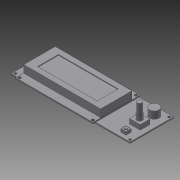
# Autodesk Inventor part: RepRapDiscount_SmartController
Saved by Autodesk Inventor 2014 (Build 180170000, 170)
## iProperties
Created: 2014-10-27
Part Number: RepRapDiscount_SmartController
Material: Generic
Document SubType Name: Modeling
Designer: ThatOtherGuy
Density: 1 g/cm^3
Appearance: Default
Author: ThatOtherGuy
Autodesk Inventor part; units mm, degrees
note: some values were not read from the file. Chosen so that the rebuilt part matches the saved one: direction of "LCD_PCB_Hole".
ref_plane "YZ Plane" through (0, 0, 0) normal (1, 0, 0) x (0, 1, 0)
ref_plane "XZ Plane" through (0, 0, 0) normal (0, 1, 0) x (-1, 0, 0)
ref_plane "XY Plane" through (0, 0, 0) normal (0, 0, 1) x (1, 0, 0)
sketch "Sketch1" plane through (0, 0, 0) normal (0, 0, 1) x (1, 0, 0)
  line L0 (0, 0) -> (150, 0)
  line L1 (150, 0) -> (150, 55)
  line L2 (150, 55) -> (0, 55)
  line L3 (0, 55) -> (0, 0)
  dimension "d0" = 150
  dimension "d1" = 55
  constraints: 8 end point, 2 parallel, 1 horizontal, 1 perpendicular
  measures "d0" distance of L1.end L2.end
  measures "d1" distance of L2.end L0.start
extrude "BackerPCB" add sketch "Sketch1" along normal blind 1.6
sketch "Sketch2" plane through (0, 0, 1.6) normal (0, 0, 1) x (1, 0, 0)
  line L0 (0, 0) -> (150, 0) projected
  line L1 (150, 0) -> (150, 55) projected
  line L2 (150, 55) -> (0, 55) projected
  line L3 (0, 55) -> (0, 0) projected
  point P0 (2.61, 52.265)
  point P1 (147.39, 52.265)
  point P2 (147.39, 2.735)
  point P3 (2.61, 2.735)
  dimension "d4" = 144.78
  dimension "d5" = 49.53
  dimension "d6" = 2.735
  dimension "d7" = 2.61
  dimension "d9" = 2.61
  dimension "d10" = 2.735
  constraints: 2 horizontal alignment, 2 vertical alignment
  measures "d4" distance of point (2.61, 52.265) point (147.39, 52.265)
  measures "d5" distance of point (2.61, 52.265) point (2.61, 2.735)
  measures "d6" distance from line of L2 point (2.61, 52.265)
  measures "d7" distance from line of L3 point (2.61, 52.265)
  measures "d9" distance from line of L1 point (147.39, 52.265)
  measures "d10" distance from line of L0 point (2.61, 2.735)
hole "BackerPCB_Holes" at (2.61, 52.265, 1.6) at (147.39, 52.265, 1.6) at (147.39, 2.735, 1.6) at (2.61, 2.735, 1.6) direction (0, 0, -1) diameter 3 end through all
sketch "Sketch3" plane through (0, 0, 0) normal (0, 0, -1) x (-1, 0, 0)
  line L0 (0, 0) -> (-150, 0) projected
  line L1 (0, 55) -> (0, 0) projected
  line L2 (0, 34.25) -> (-26, 34.25)
  line L3 (-26, 34.25) -> (-26, 7.75)
  line L4 (-26, 7.75) -> (0, 7.75)
  line L5 (0, 7.75) -> (0, 34.25)
  dimension "d18" = 26
  dimension "d19" = 26.5
  dimension "d20" = 7.75
  constraints: 8 end point, 2 parallel, 1 horizontal, 1 perpendicular, 1 point on line
  measures "d18" distance of L2.start L2.end
  measures "d19" distance of L2.end L3.end
  measures "d20" distance between parallel lines of L0 L4
extrude "SDSlot" add sketch "Sketch3" along normal blind 2.75
sketch "Sketch4" plane through (0, 0, 0) normal (0, 0, -1) x (-1, 0, 0)
  line L0 (0, 55) -> (0, 0) projected
  line L1 (-150, 55) -> (0, 55) projected
  circle A0 centre (-13, 43) radius 4.5
  dimension "d23" = 9
  dimension "d24" = 13
  dimension "d25" = 12
  constraints: 1 centre point
  measures "d23" diameter of A0
  measures "d24" distance from line of L0 A0.centre
  measures "d25" distance from line of L1 A0.centre
extrude "ContrastPot" add sketch "Sketch4" along normal blind 7.75
sketch "Sketch5" plane through (0, 0, 0) normal (0, 0, -1) x (-1, 0, 0)
  line L0 (-150, 55) -> (0, 55) projected
  line L1 (-150, 0) -> (-150, 55) projected
  line L2 (-89, 32.5) -> (-68.5, 32.5)
  line L3 (-68.5, 32.5) -> (-68.5, 23.75)
  line L4 (-68.5, 23.75) -> (-89, 23.75)
  line L5 (-89, 23.75) -> (-89, 32.5)
  line L6 (-66.1, 32.5) -> (-45.6, 32.5)
  line L7 (-45.6, 32.5) -> (-45.6, 23.75)
  line L8 (-45.6, 23.75) -> (-66.1, 23.75)
  line L9 (-66.1, 23.75) -> (-66.1, 32.5)
  dimension "d28" = 20.5
  dimension "d29" = 8.75
  dimension "d30" = 2.4
  dimension "d31" = 22.5
  dimension "d32" = 61
  constraints: 16 end point, 4 parallel, 2 equal length, 2 horizontal, 2 perpendicular, 1 collinear
  measures "d28" distance of L2.start L2.end
  measures "d29" distance of L4.end L2.start
  measures "d30" distance between parallel lines of L9 L3
  measures "d31" distance between parallel lines of L0 L2
  measures "d32" distance between parallel lines of L1 L5
extrude "Ribbons" add sketch "Sketch5" along normal blind 9
sketch "Sketch6" plane through (0, 0, 1.6) normal (0, 0, 1) x (1, 0, 0)
  line L0 (150, 0) -> (150, 55) projected
  line L1 (150, 55) -> (0, 55) projected
  circle A0 centre (136.2, 44.5) radius 6
  dimension "d35" = 13.8
  dimension "d36" = 10.5
  dimension "d37" = 12
  constraints: 1 centre point
  measures "d35" distance from line of L0 A0.centre
  measures "d36" distance from line of L1 A0.centre
  measures "d37" diameter of A0
extrude "Piezo" add sketch "Sketch6" along normal blind 9
sketch "Sketch14" plane through (0, 0, 1.6) normal (0, 0, 1) x (1, 0, 0)
  line L0 (0, 0) -> (150, 0) projected
  line L1 (150, 0) -> (150, 55) projected
  line L2 (133.65, 11.35) -> (140, 11.35)
  line L3 (140, 11.35) -> (140, 5)
  line L4 (140, 5) -> (133.65, 5)
  line L5 (133.65, 5) -> (133.65, 11.35)
  dimension "d84" = 6.35
  dimension "d85" = 5
  dimension "d86" = 10
  constraints: 8 end point, 2 parallel, 2 perpendicular, 1 horizontal
  measures "d84" distance of L2.start L2.end
  measures "d85" distance between parallel lines of L0 L4
  measures "d86" distance between parallel lines of L1 L3
extrude "Button_Base" add sketch "Sketch14" along normal blind 4
sketch "Sketch15" plane through (0, 0, 5.6) normal (0, 0, 1) x (1, 0, 0)
  line L0 (140, 11.35) -> (133.65, 11.35) projected
  line L1 (133.65, 11.35) -> (133.65, 5) projected
  circle A0 centre (136.825, 8.175) radius 2
  point P0 (0, 0)
  point P1 (136.825, 11.35)
  point P2 (133.65, 8.175)
  dimension "d89" = 4
  constraints: 2 midpoint, 1 centre point, 1 horizontal alignment, 1 vertical alignment
  measures "d89" diameter of A0
extrude "Button" add sketch "Sketch15" along normal blind 1
sketch "Sketch16" plane through (0, 0, 1.6) normal (0, 0, 1) x (1, 0, 0)
  line L0 (150, 0) -> (150, 55) projected
  line L1 (150, 55) -> (0, 55) projected
  line L2 (130, 31.5) -> (143.5, 31.5)
  line L3 (143.5, 31.5) -> (143.5, 19.5)
  line L4 (143.5, 19.5) -> (130, 19.5)
  line L5 (130, 19.5) -> (130, 31.5)
  dimension "d92" = 13.5
  dimension "d93" = 12
  dimension "d94" = 6.5
  dimension "d95" = 23.5
  constraints: 8 end point, 2 parallel, 1 horizontal, 1 perpendicular
  measures "d92" distance of L2.start L2.end
  measures "d93" distance of L4.end L2.start
  measures "d94" distance between parallel lines of L0 L3
  measures "d95" distance between parallel lines of L1 L2
extrude "Encoder_Base" add sketch "Sketch16" along normal blind 6
sketch "Sketch17" plane through (0, 0, 7.6) normal (0, 0, 1) x (1, 0, 0)
  line L0 (143.5, 31.5) -> (130, 31.5) projected
  line L1 (130, 31.5) -> (130, 19.5) projected
  circle A0 centre (136.75, 25.5) radius 3.5
  point P0 (0, 0)
  point P1 (136.75, 31.5)
  point P2 (130, 25.5)
  dimension "d98" = 7
  constraints: 2 midpoint, 1 centre point, 1 horizontal alignment, 1 vertical alignment
  measures "d98" diameter of A0
extrude "Encoder_Base_Round" add sketch "Sketch17" along normal blind 6.5
sketch "Sketch18" plane through (136.75, 25.5, 14.1) normal (0, 0, 1) x (1, 0, 0)
  circle A0 centre (0, 0) radius 3.5 projected
  circle A1 centre (0, 0) radius 3
  point P0 (-136.75, -25.5)
  dimension "d101" = 6
  constraints: 1 centre point, 1 coincident
  measures "d101" diameter of A1
extrude "Encoder_Round" add sketch "Sketch18" along normal blind 12.5 contours A1
sketch "Sketch9" plane through (0, 0, 1.6) normal (0, 0, 1) x (1, 0, 0)
  line L0 (150, 55) -> (0, 55) projected
  line L1 (0, 55) -> (0, 0) projected
  line L2 (21.59, 51.19) -> (64.77, 51.19)
  line L3 (64.77, 51.19) -> (64.77, 48.65)
  line L4 (64.77, 48.65) -> (21.59, 48.65)
  line L5 (21.59, 48.65) -> (21.59, 51.19)
  point P0 (21.59, 49.92)
  dimension "d49" = 5.08
  dimension "d50" = 2.54
  dimension "d51" = 21.59
  dimension "d52" = 43.18
  constraints: 8 end point, 2 parallel, 1 horizontal, 1 midpoint, 1 perpendicular
  measures "d49" distance from line of L0 point (21.59, 49.92)
  measures "d50" distance between parallel lines of L4 L2
  measures "d51" distance from line of L1 point (21.59, 49.92)
  measures "d52" distance of L3.end L4.end
extrude "LCD_Header" add sketch "Sketch9" along normal blind 2.54
sketch "Sketch10" plane through (0, 0, 4.14) normal (0, 0, 1) x (1, 0, 0)
  line L0 (64.77, 51.19) -> (21.59, 51.19) projected
  line L1 (21.59, 51.19) -> (21.59, 48.65) projected
  line L2 (11.43, 53.73) -> (109.22, 53.73)
  line L3 (109.22, 53.73) -> (109.22, -5.96)
  line L4 (109.22, -5.96) -> (11.43, -5.96)
  line L5 (11.43, -5.96) -> (11.43, 53.73)
  point P0 (0, 0)
  point P1 (21.59, 49.92)
  dimension "d61" = 2.54
  dimension "d62" = 59.69
  dimension "d63" = 97.79
  dimension "d64" = 10.16
  constraints: 8 end point, 2 parallel, 1 horizontal, 1 midpoint, 1 perpendicular
  measures "d61" distance between parallel lines of L2 L0
  measures "d62" distance of L4.end L2.start
  measures "d63" distance of L2.start L2.end
  measures "d64" distance between parallel lines of L5 L1
extrude "LCD_PCB" add sketch "Sketch10" along normal blind 1.6
sketch "Sketch12" plane through (0, 0, 5.74) normal (0, 0, 1) x (1, 0, 0)
  line L0 (109.22, 53.73) -> (11.43, 53.73) projected
  line L1 (11.43, 53.73) -> (11.43, -5.96) projected
  line L2 (11.43, -5.96) -> (109.22, -5.96) projected
  line L3 (109.22, -5.96) -> (109.22, 53.73) projected
  line L4 (106.68, 51.19) -> (106.68, 53.73)
  line L5 (106.68, 51.19) -> (109.22, 51.19)
  line L6 (13.97, -3.42) -> (11.43, -3.42)
  line L7 (13.97, -3.42) -> (13.97, -5.96)
  point P0 (0, 0)
  point P1 (13.97, 51.19)
  point P2 (106.68, -3.42)
  dimension "d71" = 92.71
  dimension "d72" = 54.61
  constraints: 8 end point, 4 perpendicular, 4 point on line, 2 horizontal alignment, 2 parallel, 2 vertical alignment
  measures "d71" distance of L4.start point (13.97, 51.19)
  measures "d72" distance of point (13.97, 51.19) L6.start
hole "LCD_PCB_Hole" at (13.97, 51.19, 5.74) at (106.68, 51.19, 5.74) at (106.68, -3.42, 5.74) at (13.97, -3.42, 5.74) direction (0, 0, -1) diameter 3.5 end up to surface
sketch "Sketch11" plane through (0, 0, 5.74) normal (0, 0, 1) x (1, 0, 0)
  line L0 (109.22, 53.73) -> (11.43, 53.73) projected
  line L1 (11.43, 53.73) -> (11.43, -5.96) projected
  line L2 (11.43, -5.96) -> (109.22, -5.96) projected
  line L3 (109.22, -5.96) -> (109.22, 53.73) projected
  line L4 (11.825, 43.76) -> (108.825, 43.76)
  line L5 (108.825, 43.76) -> (108.825, 4.01)
  line L6 (108.825, 4.01) -> (11.825, 4.01)
  line L7 (11.825, 4.01) -> (11.825, 43.76)
  line L8 (11.825, 43.76) -> (11.43, 43.76)
  line L9 (108.825, 43.76) -> (109.22, 43.76)
  line L10 (11.825, 43.76) -> (11.825, 53.73)
  line L11 (11.825, 4.01) -> (11.825, -5.96)
  point P0 (0, 0)
  dimension "d67" = 97
  dimension "d68" = 39.75
  constraints: 16 end point, 5 perpendicular, 4 point on line, 2 collinear, 2 parallel, 1 horizontal
  measures "d67" distance of L4.start L4.end
  measures "d68" distance of L6.end L4.start
extrude "LCD" add sketch "Sketch11" along normal blind 9.5 contours L4 L5 L6 L7
sketch "Sketch13" plane through (0, 0, 15.24) normal (0, 0, 1) x (1, 0, 0)
  line L0 (11.825, 43.76) -> (11.825, 4.01) projected
  line L1 (11.825, 4.01) -> (108.825, 4.01) projected
  line L2 (108.825, 4.01) -> (108.825, 43.76) projected
  line L3 (108.825, 43.76) -> (11.825, 43.76) projected
  line L4 (22.575, 37.135) -> (98.075, 37.135)
  line L5 (98.075, 37.135) -> (98.075, 10.635)
  line L6 (98.075, 10.635) -> (22.575, 10.635)
  line L7 (22.575, 10.635) -> (22.575, 37.135)
  line L8 (98.075, 37.135) -> (98.075, 43.76)
  line L9 (98.075, 37.135) -> (108.825, 37.135)
  line L10 (22.575, 10.635) -> (22.575, 4.01)
  line L11 (22.575, 10.635) -> (11.825, 10.635)
  point P0 (0, 0)
  dimension "d80" = 75.5
  dimension "d81" = 26.5
  constraints: 16 end point, 5 parallel, 4 perpendicular, 4 point on line, 1 horizontal
  measures "d80" distance of L4.start L4.end
  measures "d81" distance of L4.end L5.end
extrude "LCD_Inset" cut sketch "Sketch13" against normal blind 1 contours L7 L4 L5 L6
equation "\"d6\" = d10"
equation "\"d7\" = d9"
body "Solid1"
